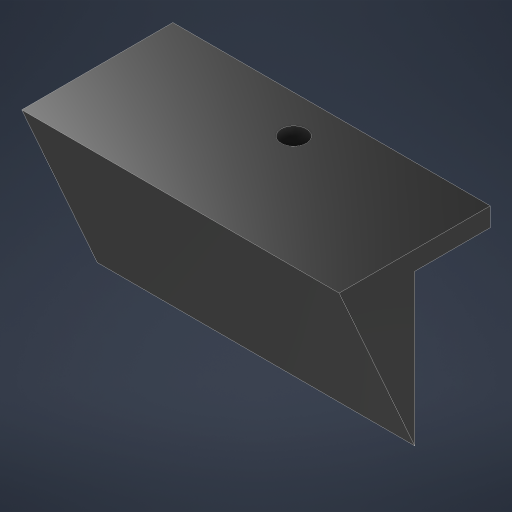
# Autodesk Inventor part: sleds v2
Saved by Autodesk Inventor 2024 (Build 280153000, 153)
## iProperties
Created: 2023-12-20
Part Number: sleds v2
Material: Generic
Document SubType Name: Modeling
Designer: elite
Density: 1 g/cm^3
Appearance: Glossy - Black
Author: elite
Autodesk Inventor part; units mm, degrees
ref_plane "YZ Plane" through (0, 0, 0) normal (1, 0, 0) x (0, 1, 0)
ref_plane "XZ Plane" through (0, 0, 0) normal (0, 1, 0) x (-1, 0, 0)
ref_plane "XY Plane" through (0, 0, 0) normal (0, 0, 1) x (1, 0, 0)
sketch "Sketch1" plane through (0, 0, 0) normal (1, 0, 0) x (0, 1, 0)
  line L0 (0, 0) -> (25.4, 0)
  line L1 (25.4, 0) -> (28.575, 0)
  line L2 (28.575, 0) -> (28.575, -12.7)
  line L3 (28.575, -12.7) -> (25.4, -12.7)
  line L4 (25.4, -12.7) -> (25.4, 0)
  line L5 (28.575, 0) -> (28.575, 12.7)
  line L6 (28.575, 12.7) -> (0, 0)
  dimension "d0" = 25.4
  dimension "d1" = 3.175
  dimension "d2" = 12.7
  dimension "d3" = 12.7
  constraints: 14 end point, 3 perpendicular, 2 point on line, 1 horizontal
  measures "d0" distance of L0.start L0.end
  measures "d1" distance of L0.end L1.end
  measures "d2" distance of L1.end L2.end
  measures "d3" distance of L1.end L5.end
extrude "Extrusion1" add sketch "Sketch1" along normal blind 53.34
sketch "Sketch2" plane through (0, 28.575, 12.7) normal (0, 1, 0) x (1, 0, 0)
  line L0 (53.34, 25.4) -> (53.34, 19.05)
  line L1 (53.34, 25.4) -> (53.34, 0) projected
  line L2 (53.34, 19.05) -> (26.67, 19.05)
  circle A0 centre (26.67, 19.05) radius 2.1082
  point P0 (0, 12.7)
  dimension "d6" = 6.35
  dimension "d7" = 26.67
  dimension "d8" = 4.2164
  constraints: 4 end point, 1 centre point, 1 coincident, 1 horizontal, 1 point on line
  measures "d6" distance of L0.start L0.end
  measures "d7" distance of L0.end L2.end
  measures "d8" diameter of A0
extrude "Extrusion2" cut sketch "Sketch2" against normal blind 43.815
body "Solid1"
